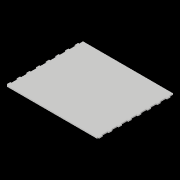
# Autodesk Inventor part: Back 2 V3
Saved by Autodesk Inventor 2018 (Build 220112000, 112)
## iProperties
Created: 2017-09-14
Part Number: Back 2 V3
Material: Generic
Document SubType Name: Modeling
Designer: gaine
Density: 1 g/cm^3
Appearance: Default
Author: gaine
Autodesk Inventor part; units mm, degrees
ref_plane "YZ Plane" through (0, 0, 0) normal (1, 0, 0) x (0, 1, 0)
ref_plane "XZ Plane" through (0, 0, 0) normal (0, 1, 0) x (-1, 0, 0)
ref_plane "XY Plane" through (0, 0, 0) normal (0, 0, 1) x (1, 0, 0)
sketch "Sketch1" plane through (0, 0, 0) normal (0, 1, 0) x (-1, 0, 0)
  line L0 (84.5044, -277.3965) -> (-445.7206, -277.3965)
  line L1 (-445.7206, -725.5287) -> (84.5044, -725.5287)
  line L2 (-445.7206, -277.3965) -> (-445.7206, -283.7465)
  line L3 (-445.7206, -283.7465) -> (-452.0706, -283.7465)
  line L4 (-452.0706, -302.7965) -> (-445.7206, -302.7965)
  line L5 (-445.7206, -302.7965) -> (-445.7206, -340.8965)
  line L6 (-445.7206, -340.8965) -> (-452.0706, -340.8965)
  line L7 (-452.0706, -359.9465) -> (-445.7206, -359.9465)
  line L8 (-445.7206, -359.9465) -> (-445.7206, -398.0465)
  line L9 (-445.7206, -398.0465) -> (-452.0706, -398.0465)
  line L10 (-452.0706, -417.0965) -> (-445.7206, -417.0965)
  line L11 (-445.7206, -417.0965) -> (-445.7206, -455.1965)
  line L12 (-445.7206, -455.1965) -> (-452.0706, -455.1965)
  line L13 (-452.0706, -474.2465) -> (-445.7206, -474.2465)
  line L14 (-445.7206, -512.3465) -> (-452.0706, -512.3465)
  line L15 (-452.0706, -531.3965) -> (-445.7206, -531.3965)
  line L16 (-445.7206, -531.3965) -> (-445.7206, -569.4965)
  line L17 (-445.7206, -569.4965) -> (-452.0706, -569.4965)
  line L18 (-452.0706, -588.5465) -> (-445.7206, -588.5465)
  line L19 (-445.7206, -588.5465) -> (-445.7206, -626.6465)
  line L20 (-445.7206, -626.6465) -> (-452.0706, -626.6465)
  line L21 (-452.0706, -645.6965) -> (-445.7206, -645.6965)
  line L22 (-445.7206, -645.6965) -> (-445.7206, -683.7965)
  line L23 (-445.7206, -683.7965) -> (-452.0706, -683.7965)
  line L24 (-452.0706, -702.8465) -> (-445.7206, -702.8465)
  line L25 (-445.7206, -702.8465) -> (-445.7206, -725.5287)
  line L26 (-452.0706, -283.7465) -> (-452.0706, -302.7965)
  line L27 (-452.0706, -340.8965) -> (-452.0706, -359.9465)
  line L28 (-452.0706, -398.0465) -> (-452.0706, -417.0965)
  line L29 (-452.0706, -455.1965) -> (-452.0706, -474.2465)
  line L30 (-452.0706, -512.3465) -> (-452.0706, -531.3965)
  line L31 (-452.0706, -569.4965) -> (-452.0706, -588.5465)
  line L32 (-452.0706, -626.6465) -> (-452.0706, -645.6965)
  line L33 (-452.0706, -683.7965) -> (-452.0706, -702.8465)
  line L34 (-445.7206, -512.3465) -> (-445.7206, -474.2465)
  line L35 (84.5044, -277.3965) -> (84.5044, -283.7465)
  line L36 (84.5044, -283.7465) -> (90.8544, -283.7465)
  line L37 (90.8544, -302.7965) -> (84.5044, -302.7965)
  line L38 (84.5044, -302.7965) -> (84.5044, -340.8965)
  line L39 (84.5044, -340.8965) -> (90.8544, -340.8965)
  line L40 (90.8544, -359.9465) -> (84.5044, -359.9465)
  line L41 (84.5044, -359.9465) -> (84.5044, -398.0465)
  line L42 (84.5044, -398.0465) -> (90.8544, -398.0465)
  line L43 (90.8544, -417.0965) -> (84.5044, -417.0965)
  line L44 (84.5044, -417.0965) -> (84.5044, -455.1965)
  line L45 (84.5044, -455.1965) -> (90.8544, -455.1965)
  line L46 (90.8544, -474.2465) -> (84.5044, -474.2465)
  line L47 (84.5044, -474.2465) -> (84.5044, -512.3465)
  line L48 (84.5044, -512.3465) -> (90.8544, -512.3465)
  line L49 (90.8544, -531.3965) -> (84.5044, -531.3965)
  line L50 (84.5044, -531.3965) -> (84.5044, -569.4965)
  line L51 (84.5044, -569.4965) -> (90.8544, -569.4965)
  line L52 (90.8544, -588.5465) -> (84.5044, -588.5465)
  line L53 (84.5044, -588.5465) -> (84.5044, -626.6465)
  line L54 (84.5044, -626.6465) -> (90.8544, -626.6465)
  line L55 (90.8544, -645.6965) -> (84.5044, -645.6965)
  line L56 (84.5044, -645.6965) -> (84.5044, -683.7965)
  line L57 (84.5044, -683.7965) -> (90.8544, -683.7965)
  line L58 (84.5044, -725.5287) -> (84.5044, -702.8465)
  line L59 (84.5044, -702.8465) -> (90.8544, -702.8465)
  line L60 (90.8544, -302.7965) -> (90.8544, -283.7465)
  line L61 (90.8544, -359.9465) -> (90.8544, -340.8965)
  line L62 (90.8544, -417.0965) -> (90.8544, -398.0465)
  line L63 (90.8544, -474.2465) -> (90.8544, -455.1965)
  line L64 (90.8544, -531.3965) -> (90.8544, -512.3465)
  line L65 (90.8544, -588.5465) -> (90.8544, -569.4965)
  line L66 (90.8544, -702.8465) -> (90.8544, -683.7965)
  line L67 (90.8544, -645.6965) -> (90.8544, -626.6465)
  line L68 (84.5044, -493.2965) -> (-445.7206, -493.2965)
  point P0 (0, 0)
  dimension "d53" = 6.35
  dimension "d54" = 38.1
  dimension "d55" = 19.05
  dimension "d56" = 19.05
  dimension "d57" = 19.05
  dimension "d58" = 38.1
  dimension "d59" = 38.1
  dimension "d60" = 19.05
  dimension "d61" = 38.1
  dimension "d62" = 19.05
  dimension "d63" = 38.1
  dimension "d64" = 19.05
  dimension "d65" = 38.1
  dimension "d66" = 19.05
  dimension "d67" = 38.1
  dimension "d68" = 19.05
  dimension "d69" = 6.35
  dimension "d70" = 6.35
  dimension "d71" = 6.35
  dimension "d72" = 6.35
  dimension "d74" = 6.35
  dimension "d75" = 6.35
  dimension "d76" = 6.35
  dimension "d94" = 22.6822
  dimension "d134" = 6.35
  dimension "d135" = 19.05
  dimension "d136" = 38.1
  dimension "d137" = 19.05
  dimension "d138" = 38.1
  dimension "d139" = 19.05
  dimension "d140" = 38.1
  dimension "d141" = 19.05
  dimension "d142" = 38.1
  dimension "d143" = 19.05
  dimension "d144" = 38.1
  dimension "d145" = 19.05
  dimension "d146" = 38.1
  dimension "d147" = 19.05
  dimension "d148" = 38.1
  dimension "d149" = 19.05
  dimension "d150" = 6.35
  dimension "d151" = 448.1322
  dimension "d152" = 542.925
  constraints: 138 end point, 22 collinear, 22 perpendicular, 16 horizontal, 15 parallel, 9 vertical, 2 midpoint
  measures "d53" distance between parallel lines of L33 L25
  measures "d54" distance between parallel lines of L23 L21
  measures "d55" distance between parallel lines of L24 L23
  measures "d56" distance between parallel lines of L21 L20
  measures "d57" distance between parallel lines of L18 L17
  measures "d58" distance between parallel lines of L20 L18
  measures "d59" distance between parallel lines of L17 L15
  measures "d60" distance between parallel lines of L15 L14
  measures "d61" distance between parallel lines of L14 L13
  measures "d62" distance between parallel lines of L13 L12
  measures "d63" distance between parallel lines of L12 L10
  measures "d64" distance between parallel lines of L10 L9
  measures "d65" distance between parallel lines of L9 L7
  measures "d66" distance between parallel lines of L7 L6
  measures "d67" distance between parallel lines of L6 L4
  measures "d68" distance between parallel lines of L4 L3
  measures "d69" distance between parallel lines of L3 L0
  measures "d70" distance between parallel lines of L5 L26
  measures "d71" distance between parallel lines of L8 L27
  measures "d72" distance between parallel lines of L11 L28
  measures "d74" distance between parallel lines of L16 L30
  measures "d75" distance between parallel lines of L19 L31
  measures "d76" distance between parallel lines of L22 L32
  measures "d94" distance between parallel lines of L1 L24
  measures "d134" distance between parallel lines of L58 L66
  measures "d135" distance between parallel lines of L57 L59
  measures "d136" distance between parallel lines of L55 L57
  measures "d137" distance between parallel lines of L54 L55
  measures "d138" distance between parallel lines of L52 L54
  measures "d139" distance between parallel lines of L51 L52
  measures "d140" distance between parallel lines of L49 L51
  measures "d141" distance between parallel lines of L48 L49
  measures "d142" distance between parallel lines of L46 L48
  measures "d143" distance between parallel lines of L45 L46
  measures "d144" distance between parallel lines of L43 L45
  measures "d145" distance between parallel lines of L42 L43
  measures "d146" distance between parallel lines of L40 L42
  measures "d147" distance between parallel lines of L39 L40
  measures "d148" distance between parallel lines of L37 L39
  measures "d149" distance between parallel lines of L36 L37
  measures "d150" distance between parallel lines of L0 L36
  measures "d151" distance between parallel lines of L0 L1
  measures "d152" distance between parallel lines of L33 L66
extrude "Extrusion3" add sketch "Sketch1" along normal blind 6.35
body "Solid3"
